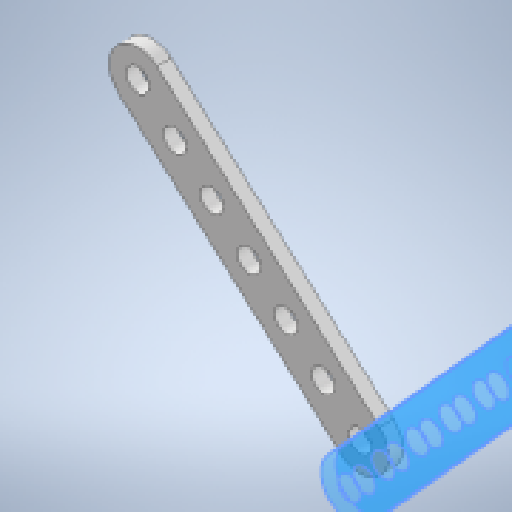
# Autodesk Inventor part: control-arm
Saved by Autodesk Inventor 2024.1 (Build 281209000, 209)
## iProperties
Created: 2025-06-12
Part Number: control-arm
Material: Generic
Document SubType Name: Modeling
Designer: iwheard
Density: 1 g/cm^3
Appearance: Default
Author: iwheard
Autodesk Inventor part; units mm, degrees
ref_plane "YZ Plane" through (0, 0, 0) normal (1, 0, 0) x (0, 1, 0)
ref_plane "XZ Plane" through (0, 0, 0) normal (0, 1, 0) x (-1, 0, 0)
ref_plane "XY Plane" through (0, 0, 0) normal (0, 0, 1) x (1, 0, 0)
sketch "Sketch1" plane through (0, 0, 0) normal (0, 0, 1) x (1, 0, 0)
  line L0 (4.2818, -5.6498) -> (9.6498, 0.2818)
  line L1 (9.6498, 0.2818) -> (-27.4231, 33.8318)
  line L2 (-27.4231, 33.8318) -> (-32.7911, 27.9001)
  line L3 (-32.7911, 27.9001) -> (4.2818, -5.6498)
  circle A0 centre (4, 0) radius 1.6 projected
  circle A1 centre (4, 0) radius 1.6
  circle A2 centre (-1.1902, 4.697) radius 1.6
  circle A3 centre (-6.3804, 9.394) radius 1.6
  circle A4 centre (-11.5706, 14.091) radius 1.6
  circle A5 centre (-16.7608, 18.788) radius 1.6
  circle A6 centre (-21.951, 23.485) radius 1.6
  circle A7 centre (-27.1413, 28.182) radius 1.6
  point P0 (0, 0)
  dimension "d0" = 8
  dimension "d1" = 4
  dimension "d2" = 4
  dimension "d5" = 7
  dimension "d10" = 4
  constraints: 8 end point, 7 centre point, 7 coincident, 2 parallel, 1 concentric, 1 perpendicular, 19 other
  measures "d0" distance between parallel lines of L1 L3
  measures "d1" distance from line of L3 A0.centre
  measures "d2" distance from line of L0 A0.centre
  measures "d5" distance of A1.centre A2.centre
  measures "d10" distance from line of A7.centre L2
extrude "Extrusion1" add sketch "Sketch1" along normal blind 2
fillet "Fillet1" radius 4 4 edges at (-32.7911, 27.9001, 1) (-27.4231, 33.8318, 1) (4.2818, -5.6498, 1) (9.6498, 0.2818, 1)
equation "\"d1\" = 0.5 * d0"
body "Solid1"
